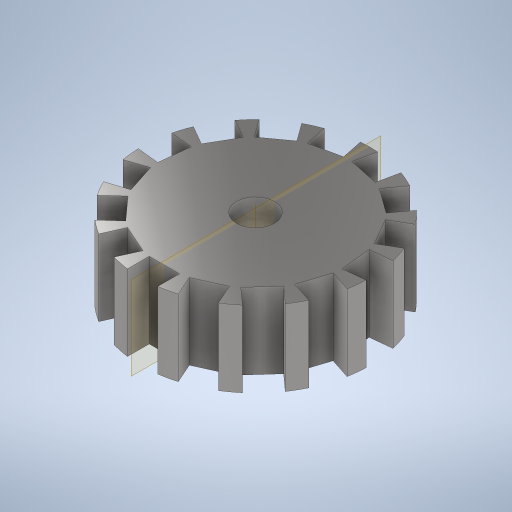
# Autodesk Inventor part: malare
Saved by Autodesk Inventor 2023 (Build 270158000, 158)
## iProperties
Created: 2022-11-26
Part Number: malare
Material: Steel, Cast
Document SubType Name: Modeling
Designer: abdul
Density: 7.85 g/cm^3
Appearance: Semi-Polished
Author: abdul
Autodesk Inventor part; units mm, degrees
ref_plane "XY Plane" through (0, 0, 0) normal (0, 0, 1) x (1, 0, 0)
sketch "Sketch1" plane through (0, 0, 0) normal (0, 1, 0) x (-1, 0, 0)
  circle A0 centre (0, 0) radius 15
  dimension "d0" = 30
  constraints: 1 centre point, 1 coincident
  measures "d0" diameter of A0
ref_plane "Work Plane1" through (0, 10, 0) normal (0, 1, 0) x (-1, 0, 0)
extrude "Extrusion1" add sketch "Sketch1" along normal blind 10
sketch "Sketch2" plane through (0, 10, 0) normal (0, 1, 0) x (1, 0, 0)
  line L0 (2, -22) -> (-2, -22)
  line L1 (-2, -22) -> (-2, -12)
  line L2 (-2, -12) -> (2, -12)
  line L3 (2, -12) -> (2, -22)
  circle A0 centre (0, 0) radius 15 projected
  point P0 (0, -12)
  dimension "d4" = 4
  dimension "d5" = 10
  dimension "d6" = 12
  constraints: 8 end point, 2 parallel, 1 horizontal, 1 midpoint, 1 perpendicular, 1 vertical alignment
  measures "d4" distance of L1.end L2.end
  measures "d5" distance of L0.end L1.end
  measures "d6" distance of point (0, -12) A0.centre
extrude "Extrusion2" cut sketch "Sketch2" against normal blind 10 contours L0 L1 A0 L3 | A0 L1 L2 L3 picked at (-0.2228, -12.995)
pattern_circular "Circular Pattern1" count 15 over 360 about axis through (0, 0, 0) along (0, 1, 0) of "Extrusion2"
sketch "Sketch6" plane through (0, 10, 0) normal (0, 1, 0) x (1, 0, 0)
  circle A0 centre (0, 0) radius 2.5
  dimension "d24" = 5
  constraints: 1 centre point, 1 coincident
  measures "d24" diameter of A0
extrude "Extrusion6" cut sketch "Sketch6" against normal blind 10
chamfer "Chamfer1" distance 1 angle 45 1 edges at (-2.5, 0, 0)
body "Solid1"
